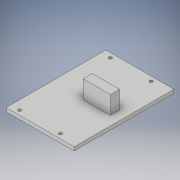
# Autodesk Inventor part: Slider
Saved by Autodesk Inventor 2019 (Build 230136000, 136)
## iProperties
Created: 2020-04-04
Part Number: Slider
Material: Generic
Document SubType Name: Modeling
Designer: james
Density: 1 g/cm^3
Appearance: Default
Author: james
Autodesk Inventor part; units mm, degrees
ref_plane "YZ Plane" through (0, 0, 0) normal (1, 0, 0) x (0, 1, 0)
ref_plane "XZ Plane" through (0, 0, 0) normal (0, 1, 0) x (-1, 0, 0)
ref_plane "XY Plane" through (0, 0, 0) normal (0, 0, 1) x (1, 0, 0)
sketch "Sketch1" plane through (0, 0, 0) normal (0, 1, 0) x (-1, 0, 0)
  line L0 (56.2338, 50.9905) -> (-39.0162, 50.9905)
  line L1 (-39.0162, 50.9905) -> (-39.0162, -88.7095)
  line L2 (-39.0162, -88.7095) -> (56.2338, -88.7095)
  line L3 (56.2338, -88.7095) -> (56.2338, 50.9905)
  point P0 (0, 0)
  dimension "d0" = 139.7
  dimension "d1" = 95.25
  constraints: 8 end point, 2 parallel, 1 horizontal, 1 perpendicular
  measures "d0" distance of L0.end L1.end
  measures "d1" distance of L0.start L0.end
extrude "Extrusion1" add sketch "Sketch1" along normal blind 5.08
sketch "Sketch2" plane through (0, 5.08, 0) normal (0, 1, 0) x (1, 0, 0)
  line L0 (-56.2338, -50.9905) -> (39.0162, -50.9905) projected
  line L1 (39.0162, 88.7095) -> (-56.2338, 88.7095) projected
  line L2 (-56.2338, 88.7095) -> (-56.2338, -50.9905) projected
  point P0 (0, 0)
  point P1 (-43.5338, -44.6405)
  point P2 (13.6162, -44.6405)
  point P3 (13.6162, 82.3595)
  point P4 (-43.5338, 82.3595)
  dimension "d4" = 0
  dimension "d5" = 6.35
  dimension "d6" = 0
  dimension "d7" = 6.35
  dimension "d8" = 0
  dimension "d9" = 0
  dimension "d10" = 12.7
  dimension "d11" = 57.15
  measures "d4" vertical distance of point (13.616, -44.641) point (-43.534, -44.641)
  measures "d5" distance from line of L0 point (13.616, -44.641)
  measures "d6" vertical distance of point (-43.534, 82.359) point (13.616, 82.359)
  measures "d7" distance from line of L1 point (-43.534, 82.359)
  measures "d8" horizontal distance of point (-43.534, 82.359) point (-43.534, -44.641)
  measures "d9" horizontal distance of point (13.616, -44.641) point (13.616, 82.359)
  measures "d10" distance from line of L2 point (-43.534, -44.641)
  measures "d11" distance of point (13.616, -44.641) point (-43.534, -44.641)
hole "Hole1" at (-43.5338, 5.08, 44.6405) at (13.6162, 5.08, 44.6405) at (13.6162, 5.08, -82.3595) at (-43.5338, 5.08, -82.3595) direction (0, -1, 0) diameter 4.4958 end through all clearance for "Flat Head Machine Screw (82)" size "#8" standard "Ansi Unified Screw Threads"
sketch "Sketch3" plane through (0, 5.08, 0) normal (0, 1, 0) x (1, 0, 0)
  line L0 (-11.7838, 12.5095) -> (26.3162, 12.5095)
  line L1 (26.3162, 12.5095) -> (26.3162, 25.2095)
  line L2 (26.3162, 25.2095) -> (-11.7838, 25.2095)
  line L3 (-11.7838, 25.2095) -> (-11.7838, 12.5095)
  line L4 (39.0162, 88.7095) -> (-56.2338, 88.7095) projected
  line L5 (-56.2338, -50.9905) -> (39.0162, -50.9905) projected
  line L6 (39.0162, -50.9905) -> (39.0162, 88.7095) projected
  point P0 (0, 0)
  dimension "d19" = 12.7
  dimension "d20" = 63.5
  dimension "d21" = 63.5
  dimension "d22" = 12.7
  dimension "d23" = 38.1
  constraints: 8 end point, 2 parallel, 1 horizontal, 1 perpendicular
  measures "d19" distance of L2.end L0.start
  measures "d20" distance between parallel lines of L4 L2
  measures "d21" distance between parallel lines of L5 L0
  measures "d22" distance between parallel lines of L6 L1
  measures "d23" distance between parallel lines of L1 L3
extrude "Extrusion2" add sketch "Sketch3" along normal blind 25.4
body "Solid1"
